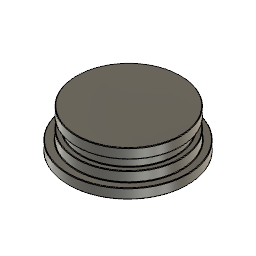
EB (Autodesk Fusion 360 design; units mm, degrees)
part number: 2026-04-20-11-05-31-891
Autodesk Fusion 360 part; units mm, degrees
sketch "Sketch1" plane through (0, 0, 0) normal (0, 0, 1) x (1, 0, 0)
  circle A0 centre (-0.7262, 0) radius 60
  dimension "d1" = 120
  measures "d1" diameter of A0
extrude "Extrude1" add sketch "Sketch1" along normal blind 10
sketch "Sketch2" plane through (0, 0, 10) normal (0, 0, 1) x (-1, 0, 0)
  circle A0 centre (0.7262, 0) radius 60
  circle A1 centre (0, 0) radius 52.5
  dimension "d4" = 105
  constraint coincident A1.centre origin
  measures "d4" diameter of A1
extrude "Extrude2" add sketch "Sketch2" along normal blind 10 contours A1
sketch "Sketch3" plane through (0, 0, 20) normal (0, 0, 1) x (-1, 0, 0)
  circle A0 centre (0, 0) radius 52.5
  circle A1 centre (0, 0) radius 47.5
  dimension "d7" = 95
  constraint coincident A0.centre A1.centre
  measures "d7" diameter of A1
extrude "Extrude3" add sketch "Sketch3" along normal blind 10 contours A1
sketch "Sketch4" plane through (0, 0, 30) normal (0, 0, 1) x (-1, 0, 0)
  circle A0 centre (0, 0) radius 47.5
  circle A1 centre (0, 0) radius 52.5
  dimension "d10" = 105
  constraint coincident A0.centre A1.centre
  measures "d10" diameter of A1
extrude "Extrude4" add sketch "Sketch4" along normal blind 10 contours A0 | A1
fillet "Fillet1" radius 0.5 8 edges at (-56.6659, -21.6969, 10) (48.9472, 18.9848, 20) (44.2855, -17.1767, 20) (48.9472, 18.9848, 30) (44.2855, 17.1767, 30) (48.9472, 18.9848, 40) (48.9472, -18.9848, 10) (-56.6659, -21.6969, 0)
